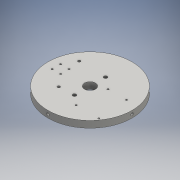
# Autodesk Inventor part: outsideCover
Saved by Autodesk Inventor 2016 (Build 200138000, 138)
## iProperties
Created: 2016-10-27
Part Number: outsideCover
Material: 一般
Document SubType Name: Modeling
Designer: Daisuke
Density: 1 g/cm^3
Appearance: 既定
Author: Daisuke
Autodesk Inventor part; units mm, degrees
sketch "スケッチ1" plane through (0, 0, 0) normal (0, 0, 1) x (1, 0, 0)
  circle A0 centre (0, 0) radius 50
  dimension "d0" = 100
  constraints: 1 centre point, 1 coincident
  measures "d0" diameter of A0
extrude "押し出し1" add sketch "スケッチ1" along normal blind 8
ref_plane "作業平面1" through (50, 0, 0) normal (1, 0, 0) x (0, 1, 0)
ref_plane "作業平面2" through (-50, 0, 0) normal (1, 0, 0) x (0, 1, 0)
ref_plane "作業平面3" through (0, 50, 0) normal (0, 1, 0) x (-1, 0, 0)
ref_plane "作業平面4" through (0, -50, 0) normal (0, 1, 0) x (-1, 0, 0)
sketch "スケッチ2" plane through (50, 0, 0) normal (1, 0, 0) x (0, 1, 0)
  line L0 (0, 0) -> (0, 4) construction
  circle A0 centre (0, 4) radius 1.5
  dimension "d7" = 4
  dimension "d8" = 3
  constraints: 2 end point, 1 centre point, 1 coincident, 1 vertical
  measures "d7" distance of L0.start L0.end
  measures "d8" diameter of A0
extrude "押し出し2" cut sketch "スケッチ2" against normal blind 5
sketch "スケッチ3" plane through (-50, 0, 0) normal (1, 0, 0) x (0, 1, 0)
  line L0 (0, 0) -> (0, 4) construction
  circle A0 centre (0, 4) radius 1.5
  dimension "d11" = 4
  dimension "d12" = 3
  constraints: 2 end point, 1 centre point, 1 coincident, 1 vertical
  measures "d11" distance of L0.start L0.end
  measures "d12" diameter of A0
extrude "押し出し3" cut sketch "スケッチ3" along normal blind 5
sketch "スケッチ4" plane through (0, 50, 0) normal (0, 1, 0) x (-1, 0, 0)
  line L0 (0, 0) -> (0, 4) construction
  circle A0 centre (0, 4) radius 1.5
  dimension "d15" = 4
  dimension "d16" = 3
  constraints: 2 end point, 1 centre point, 1 coincident, 1 vertical
  measures "d15" distance of L0.start L0.end
  measures "d16" diameter of A0
extrude "押し出し4" cut sketch "スケッチ4" against normal blind 5
sketch "スケッチ5" plane through (0, -50, 0) normal (0, 1, 0) x (-1, 0, 0)
  line L0 (0, 0) -> (0, 4) construction
  circle A0 centre (0, 4) radius 1.5
  dimension "d19" = 4
  dimension "d20" = 3
  constraints: 2 end point, 1 centre point, 1 coincident, 1 vertical
  measures "d19" distance of L0.start L0.end
  measures "d20" diameter of A0
extrude "押し出し5" cut sketch "スケッチ5" along normal blind 5
thread "ねじ1" size "M3x0.5" class "6H" standard "ANSI Metric M Profile" full length
thread "ねじ2" size "M3x0.5" class "6H" standard "ANSI Metric M Profile" full length
thread "ねじ3" size "M3x0.5" class "6H" standard "ANSI Metric M Profile" full length
thread "ねじ4" size "M3x0.5" class "6H" standard "ANSI Metric M Profile" full length
sketch "スケッチ8" plane through (0, 0, 8) normal (0, 0, 1) x (1, 0, 0)
  line L0 (0, 0) -> (0, 18.5) construction
  line L1 (0, 0) -> (0, -18.5) construction
  circle A0 centre (0, 18.5) radius 2
  circle A1 centre (0, -18.5) radius 2
  circle A2 centre (0, 0) radius 6.5
  dimension "d62" = 18.5
  dimension "d63" = 18.5
  dimension "d64" = 4
  dimension "d65" = 4
  dimension "d66" = 13
  constraints: 4 end point, 3 centre point, 3 coincident
  measures "d62" distance of point (0, 0) L0.end
  measures "d63" distance of point (0, 0) L1.end
  measures "d64" diameter of A0
  measures "d65" diameter of A1
  measures "d66" diameter of A2
extrude "押し出し7" cut sketch "スケッチ8" against normal blind 8
thread "ねじ7" size "M4x0.7" class "6H" standard "ANSI Metric M Profile" full length
thread "ねじ8" size "M4x0.7" class "6H" standard "ANSI Metric M Profile" full length
sketch "スケッチ9" plane through (0, 0, 8) normal (0, 0, 1) x (1, 0, 0)
  line L0 (0, 0) -> (25, 0) construction
  line L1 (25, 0) -> (25, -1) construction
  line L2 (25, 0) -> (25, 7.5) construction
  circle A0 centre (36, 7.5) radius 1
  line L3 (36, 7.5) -> (14, 7.5) construction
  circle A1 centre (14, 7.5) radius 1
  line L4 (25, -1) -> (25, -10) construction
  line L5 (25, -10) -> (25, -28) construction
  circle A2 centre (11.5, -28) radius 1
  line L6 (25, 0) -> (9, 0) construction
  line L7 (9, 0) -> (9, -31) construction
  line L8 (9, -31) -> (41, -31) construction
  line L9 (41, -31) -> (41, 0) construction
  line L10 (25, 0) -> (25, 12) construction
  line L11 (14.417, 12) -> (35.583, 12) construction
  arc A3 (14.757, 12.2915) -> (9, 0) centre (25, 0) ccw construction
  arc A4 (41, 0) -> (35.583, 12) centre (25, 0) ccw construction
  line L12 (11.5, -28) -> (38.5, -28) construction
  circle A5 centre (38.5, -28) radius 1
  dimension "d92" = 25
  dimension "d103" = 7.5
  dimension "d105" = 2
  dimension "d108" = 2
  dimension "d117" = 2
  dimension "d129" = 16
  dimension "d130" = 31
  dimension "d131" = 32
  dimension "d134" = 22
  dimension "d146" = 28
  dimension "d147" = 27
  dimension "d148" = 2
  constraints: 26 end point, 6 centre point, 5 point on circle, 5 vertical, 4 coincident, 3 horizontal, 3 perpendicular, 1 midpoint, 1 point on line
  measures "d92" distance of L0.start L0.end
  measures "d103" distance of L0.end L2.end
  measures "d105" diameter of A0
  measures "d108" diameter of A1
  measures "d117" diameter of A2
  measures "d129" distance of L0.end L6.end
  measures "d130" distance of L6.end L7.end
  measures "d131" distance of L7.end L8.end
  measures "d134" distance of L3.start L3.end
  measures "d146" distance of L5.end L0.end
  measures "d147" distance of L12.start L12.end
  measures "d148" diameter of A5
sketch "スケッチ10" plane through (0, 0, 8) normal (0, 0, 1) x (1, 0, 0)
  line L0 (0, 0) -> (-25, 0) construction
  line L1 (-35.65, 22.85) -> (-14.35, 22.85) construction
  line L2 (-14.35, 22.85) -> (-14.35, -22.85) construction
  line L3 (-14.35, -22.85) -> (-35.65, -22.85) construction
  line L4 (-35.65, -22.85) -> (-35.65, 22.85) construction
  line L5 (-35.65, 22.85) -> (-14.35, -22.85) construction
  line L6 (-14.35, 22.85) -> (-35.65, -22.85) construction
  line L7 (-35.65, 22.85) -> (-32.15, 22.85) construction
  line L8 (-32.15, 22.85) -> (-32.15, 19.35) construction
  line L9 (-32.15, 19.35) -> (-35.65, 19.35) construction
  line L10 (-35.65, 19.35) -> (-35.65, 22.85) construction
  line L11 (-14.35, -22.85) -> (-17.85, -22.85) construction
  line L12 (-17.85, -22.85) -> (-17.85, -19.35) construction
  line L13 (-17.85, -19.35) -> (-14.35, -19.35) construction
  line L14 (-14.35, -19.35) -> (-14.35, -22.85) construction
  circle A0 centre (-32.15, 19.35) radius 1.5
  circle A1 centre (-17.85, -19.35) radius 1.5
  dimension "d135" = 25
  dimension "d136" = 21.3
  dimension "d137" = 45.7
  dimension "d138" = 3.5
  dimension "d139" = 3.5
  dimension "d140" = 3.5
  dimension "d141" = 3.5
  dimension "d142" = 3
  dimension "d143" = 3
  constraints: 30 end point, 6 parallel, 4 horizontal, 3 perpendicular, 2 centre point, 2 coincident, 2 midpoint
  measures "d135" distance of L0.start L0.end
  measures "d136" distance of L2.end L3.end
  measures "d137" distance of L1.end L2.end
  measures "d138" distance of L8.end L9.end
  measures "d139" distance of L7.end L8.end
  measures "d140" distance of L12.end L13.end
  measures "d141" distance of L11.end L12.end
  measures "d142" diameter of A0
  measures "d143" diameter of A1
extrude "押し出し10" cut sketch "スケッチ10" against normal blind 8
extrude "押し出し11" cut sketch "スケッチ9" against normal blind 8
sketch "スケッチ13" plane through (0, 0, 8) normal (0, 0, 1) x (1, 0, 0)
  line L0 (0, 0) -> (-35, 0) construction
  line L1 (-40, 5) -> (-30, 5) construction
  line L2 (-30, 5) -> (-30, -5) construction
  line L3 (-30, -5) -> (-40, -5) construction
  line L4 (-40, -5) -> (-40, 5) construction
  line L5 (-40, 5) -> (-30, -5) construction
  line L6 (-30, 5) -> (-40, -5) construction
  circle A0 centre (-30, 5) radius 1
  circle A1 centre (-30, -5) radius 1
  circle A2 centre (-40, 5) radius 1
  circle A3 centre (-40, -5) radius 1
  dimension "d151" = 35
  dimension "d152" = 10
  dimension "d153" = 10
  dimension "d154" = 2
  dimension "d155" = 2
  dimension "d156" = 2
  dimension "d157" = 2
  constraints: 14 end point, 4 centre point, 4 coincident, 2 horizontal, 2 midpoint, 2 parallel, 1 perpendicular
  measures "d151" distance of L0.start L0.end
  measures "d152" distance of L2.end L3.end
  measures "d153" distance of L1.end L2.end
  measures "d154" diameter of A0
  measures "d155" diameter of A1
  measures "d156" diameter of A2
  measures "d157" diameter of A3
extrude "押し出し12" cut sketch "スケッチ13" against normal blind 8
